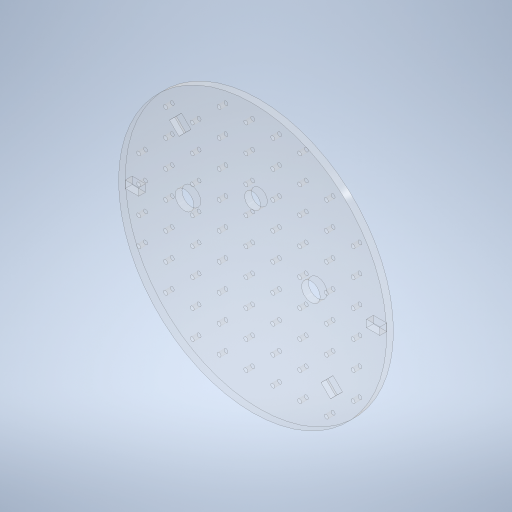
# Autodesk Inventor part: Top plate
Saved by Autodesk Inventor 2023.2 (Build 272271000, 271)
## iProperties
Created: 2024-08-12
Part Number: Top plate
Material: Polycarbonate, Clear
Document SubType Name: Modeling
Designer: PC
Density: 1.2 g/cm^3
Appearance: Polycarbonate - Clear
Author: PC
Autodesk Inventor part; units mm, degrees
ref_plane "YZ Plane" through (0, 0, 0) normal (1, 0, 0) x (0, 1, 0)
ref_plane "XZ Plane" through (0, 0, 0) normal (0, 1, 0) x (-1, 0, 0)
ref_plane "XY Plane" through (0, 0, 0) normal (0, 0, 1) x (1, 0, 0)
sketch "Sketch1" plane through (0, 0, 0) normal (0, 0, 1) x (1, 0, 0)
  line L0 (-45, -45) -> (45, -45) construction
  line L1 (-25, 25) -> (25, 25) construction
  circle A0 centre (-5, 65) radius 1.5
  circle A1 centre (-25, 65) radius 1.5
  circle A2 centre (-5, 45) radius 1.5
  circle A3 centre (-25, 45) radius 1.5
  circle A4 centre (-45, 65) radius 1.5
  circle A5 centre (-45, 45) radius 1.5
  line L2 (5, 5) -> (-5, 5) construction
  circle A6 centre (-5, 25) radius 1.5
  circle A7 centre (-5, -15) radius 1.5
  circle A8 centre (15, 25) radius 1.5
  circle A9 centre (15, 5) radius 1.5
  line L3 (-5, 5) -> (-5, -5) construction
  circle A10 centre (-5, 5) radius 1.5
  line L4 (-45, 45) -> (-45, -45) construction
  circle A11 centre (0, 37) radius 6
  line L5 (25, 25) -> (25, -25) construction
  line L6 (-65, -65) -> (-65, 65) construction
  line L7 (45, 45) -> (-45, 45) construction
  line L8 (65, -65) -> (-65, -65) construction
  line L9 (-65, 65) -> (65, 65) construction
  circle A12 centre (0, 0) radius 100
  line L10 (65, -65) -> (-65, 65) construction
  line L11 (-65, -65) -> (65, 65) construction
  line L12 (45, -45) -> (45, 45) construction
  line L13 (65, 65) -> (65, -65) construction
  circle A13 centre (35, 25) radius 1.5
  circle A14 centre (15, 45) radius 1.5
  circle A15 centre (55, 25) radius 1.5
  circle A16 centre (35, 45) radius 1.5
  circle A17 centre (15, 65) radius 1.5
  circle A18 centre (35, 65) radius 1.5
  circle A19 centre (55, 45) radius 1.5
  circle A20 centre (55, 65) radius 1.5
  circle A21 centre (75, 25) radius 1.5
  circle A22 centre (75, 45) radius 1.5
  circle A23 centre (-65, -35) radius 1.5
  circle A24 centre (-85, -35) radius 1.5
  circle A25 centre (-25, -35) radius 1.5
  circle A26 centre (-45, -35) radius 1.5
  circle A27 centre (-65, -55) radius 1.5
  circle A28 centre (-45, -55) radius 1.5
  circle A29 centre (-25, -55) radius 1.5
  circle A30 centre (75, 5) radius 1.5
  line L14 (0, 0) -> (87, 0) construction
  circle A31 centre (55, 5) radius 1.5
  circle A32 centre (35, 5) radius 1.5
  circle A33 centre (43.5, 0) radius 7
  line L15 (5, -5) -> (5, 5) construction
  circle A34 centre (-25, -15) radius 1.5
  circle A35 centre (-50.7887, 12.0679) radius 7
  circle A36 centre (-45, -15) radius 1.5
  line L16 (-25, -25) -> (-25, 25) construction
  circle A37 centre (-65, 65) radius 1.5
  circle A38 centre (-65, 45) radius 1.5
  circle A39 centre (-65, 25) radius 1.5
  circle A40 centre (-65, 5) radius 1.5
  circle A41 centre (-65, -15) radius 1.5
  circle A42 centre (-85, -15) radius 1.5
  circle A43 centre (-45, 5) radius 1.5
  circle A44 centre (-25, 5) radius 1.5
  circle A45 centre (-85, 5) radius 1.5
  circle A46 centre (-25, 25) radius 1.5
  circle A47 centre (-45, 25) radius 1.5
  circle A48 centre (-85, 25) radius 1.5
  line L17 (-5, -5) -> (5, -5) construction
  circle A49 centre (15, -15) radius 1.5
  circle A50 centre (35, -15) radius 1.5
  circle A51 centre (55, -15) radius 1.5
  circle A52 centre (75, -15) radius 1.5
  circle A53 centre (35, -35) radius 1.5
  circle A54 centre (55, -35) radius 1.5
  circle A55 centre (35, -55) radius 1.5
  circle A56 centre (55, -55) radius 1.5
  circle A57 centre (75, -35) radius 1.5
  circle A58 centre (75, -55) radius 1.5
  line L18 (25, -25) -> (-25, -25) construction
  circle A59 centre (-5, -55) radius 1.5
  circle A60 centre (15, -55) radius 1.5
  circle A61 centre (15, -35) radius 1.5
  circle A62 centre (-5, -35) radius 1.5
  line L19 (-25, 65) -> (-25, 90.4195) construction
  circle A63 centre (-25, 85) radius 1.5
  circle A64 centre (-5, 85) radius 1.5
  circle A65 centre (15, 85) radius 1.5
  circle A66 centre (35, 85) radius 1.5
  circle A67 centre (-45, -75) radius 1.5
  circle A68 centre (-25, -75) radius 1.5
  circle A69 centre (-5, -75) radius 1.5
  circle A70 centre (15, -75) radius 1.5
  circle A71 centre (35, -75) radius 1.5
  circle A72 centre (55, -75) radius 1.5
  point P0 (-14.7887, 30.5879)
  point P1 (-34.7887, 111.9312)
  point P2 (-39.9487, 111.9312)
  point P3 (-25, 0)
  dimension "d56" = 200
  dimension "d57" = 130
  dimension "d58" = 20
  dimension "d59" = 20
  dimension "d60" = 20
  dimension "d61" = 3
  dimension "d62" = 20
  dimension "d63" = 20
  dimension "d64" = 20
  dimension "d65" = 20
  dimension "d66" = 20
  dimension "d67" = 20
  dimension "d68" = 20
  dimension "d69" = 20
  dimension "d70" = 20
  dimension "d71" = 20
  dimension "d72" = 20
  dimension "d73" = 20
  dimension "d74" = 20
  dimension "d75" = 12
  dimension "d76" = 37
  dimension "d78" = 14
  dimension "d79" = 14
  dimension "d80" = 43.5
  dimension "d81" = 20
  dimension "d82" = 20
  dimension "d83" = 20
  dimension "d84" = 20
  dimension "d85" = 20
  dimension "d86" = 20
  dimension "d87" = 20
  dimension "d88" = 20
  dimension "d89" = 20
  dimension "d90" = 20
  constraints: 73 centre point, 40 end point, 14 horizontal, 8 parallel, 4 midpoint, 4 perpendicular, 3 coincident, 3 vertical, 127 other
  measures "d56" diameter of A12
  measures "d57" distance of L8.end L6.end
  measures "d58" distance between parallel lines of L9 L7
  measures "d59" distance between parallel lines of L7 L1
  measures "d60" distance between parallel lines of L1 L2
  measures "d61" diameter of A37
  measures "d62" distance of A37.centre A4.centre
  measures "d63" distance of A37.centre A38.centre
  measures "d64" distance of A38.centre A5.centre
  measures "d65" distance of A39.centre A47.centre
  measures "d66" distance of A40.centre A43.centre
  measures "d67" distance of A39.centre A48.centre
  measures "d68" distance of A40.centre A45.centre
  measures "d69" distance of A41.centre A42.centre
  measures "d70" distance of A41.centre A36.centre
  measures "d71" distance of A23.centre A24.centre
  measures "d72" distance of A23.centre A26.centre
  measures "d73" distance of A27.centre A28.centre
  measures "d74" distance of A19.centre A22.centre
  measures "d75" diameter of A11
  measures "d76" distance of point (0, 0) A11.centre
  measures "d78" diameter of A35
  measures "d79" diameter of A33
  measures "d80" distance of point (0, 0) A33.centre
  measures "d81" distance of L19.start A63.centre
  measures "d82" distance of A0.centre A64.centre
  measures "d83" distance of A17.centre A65.centre
  measures "d84" distance of A18.centre A66.centre
  measures "d85" distance of A28.centre A67.centre
  measures "d86" distance of A29.centre A68.centre
  measures "d87" distance of A59.centre A69.centre
  measures "d88" distance of A60.centre A70.centre
  measures "d89" distance of A55.centre A71.centre
  measures "d90" distance of A56.centre A72.centre
extrude "Extrusion1" add sketch "Sketch1" along normal blind 5.1
sketch "Sketch2" plane through (0, 0, 5.1) normal (0, 0, 1) x (1, 0, 0)
  line L0 (-84.9998, -2.58) -> (-94.9998, -2.58)
  line L1 (-94.9998, -2.58) -> (-94.9998, 2.92)
  line L2 (-94.9998, 2.92) -> (-84.9998, 2.92)
  line L3 (-84.9998, 2.92) -> (-84.9998, -2.58)
  line L4 (-84.9998, -2.58) -> (-94.9998, 2.92) construction
  line L5 (-94.9998, -2.58) -> (-84.9998, 2.92) construction
  line L6 (0, 0) -> (0, -10.4445) construction
  line L7 (84.9998, -2.58) -> (94.9998, -2.58)
  line L8 (94.9998, -2.58) -> (94.9998, 2.92)
  line L9 (94.9998, 2.92) -> (84.9998, 2.92)
  line L10 (84.9998, 2.92) -> (84.9998, -2.58)
  line L11 (84.9998, -2.58) -> (94.9998, 2.92) construction
  line L12 (94.9998, -2.58) -> (84.9998, 2.92) construction
  point P0 (-89.9998, 0.17)
  point P1 (89.9998, 0.17)
  dimension "d107" = 10
  dimension "d108" = 5.5
  dimension "d109" = 2.58
  dimension "d110" = 90
  constraints: 26 end point, 5 symmetric about line, 2 midpoint, 2 parallel, 1 horizontal, 1 perpendicular, 1 vertical
  measures "d107" distance of L1.end L2.end
  measures "d108" distance of L0.end L1.end
  measures "d109" distance from line of L6.start L0
  measures "d110" distance of L6.start point (-90, 0.17)
extrude "Extrusion2" cut sketch "Sketch2" against normal blind 10
sketch "Sketch3" plane through (0, 0, 5.1) normal (0, 0, 1) x (1, 0, 0)
  circle A0 centre (0, 0) radius 100 projected
  line L0 (0, 0) -> (-46.9056, 0) construction
  line L1 (0, 0) -> (-26.1892, -26.1892) construction
  line L2 (-58.0927, 61.9818) -> (-51.0885, 54.9776)
  line L3 (0, 0) -> (-61.6815, 61.6815) construction
  line L4 (-61.9818, 58.0927) -> (-54.9776, 51.0885)
  line L5 (-58.0927, 61.9818) -> (-61.9818, 58.0927)
  line L6 (-54.9776, 51.0885) -> (-51.0885, 54.9776)
  line L7 (61.9818, -58.0927) -> (54.9776, -51.0885)
  line L8 (0, 0) -> (61.6815, -61.6815) construction
  line L9 (58.0927, -61.9818) -> (51.0885, -54.9776)
  line L10 (61.9818, -58.0927) -> (58.0927, -61.9818)
  line L11 (51.0885, -54.9776) -> (54.9776, -51.0885)
  point P0 (-30.8407, 30.8407)
  point P1 (-53.5003, 53.5003)
  point P2 (-54.5906, 58.4797)
  point P3 (-58.4797, 54.5906)
  point P4 (53.5003, -53.5003)
  point P5 (58.4797, -54.5906)
  point P6 (54.5906, -58.4797)
  dimension "d117" = 45
  dimension "d123" = 45
  dimension "d126" = 80
  dimension "d127" = 80
  dimension "d128" = 2.75
  dimension "d129" = 2.75
  dimension "d130" = 75
  constraints: 24 end point, 8 symmetric about line, 4 midpoint, 2 parallel, 2 point on line, 1 horizontal, 1 perpendicular
  measures "d117" angle of L1 L0
  measures "d123" angle of L0 L3
  measures "d126" distance of point (0, 0) point (-54.591, 58.48)
  measures "d127" distance of point (0, 0) point (-58.48, 54.591)
  measures "d128" distance from line of L3 point (-58.48, 54.591)
  measures "d129" distance from line of L3 point (-54.591, 58.48)
  measures "d130" distance from line of point (0, 0) L6
extrude "Extrusion3" cut sketch "Sketch3" against normal blind 10 contours L2 L6 L4 L5 | L10 L9 L11 L7
body "Solid1"
